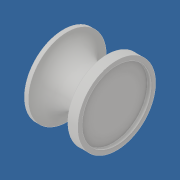
# Autodesk Inventor part: Brennersockel
Saved by Autodesk Inventor 2018 (Build 220112000, 112)
## iProperties
Created: 2018-10-20
Part Number: Brennersockel
Material: Generisch
Document SubType Name: Modeling
Designer: M.Knabel
Density: 1 g/cm^3
Appearance: Vorgabe
Author: M.Knabel
Autodesk Inventor part; units mm, degrees
ref_plane "YZ Plane" through (0, 0, 0) normal (1, 0, 0) x (0, 1, 0)
ref_plane "XZ Plane" through (0, 0, 0) normal (0, 1, 0) x (-1, 0, 0)
ref_plane "XY Plane" through (0, 0, 0) normal (0, 0, 1) x (1, 0, 0)
sketch "Skizze1" plane through (0, 0, 0) normal (0, 0, 1) x (1, 0, 0)
  line L0 (-5.4, 0) -> (32.4, 0) projected
  line L1 (0, -3.95) -> (0, 23.7) projected
  line L2 (0, 0) -> (0, 19.75)
  line L3 (2, 19.75) -> (0, 19.75)
  arc A0 (2, 19.75) -> (22, 19.75) centre (12, 19.75) ccw
  line L4 (22, 19.75) -> (27, 19.75)
  line L5 (27, 19.75) -> (27, 17.5)
  line L6 (27, 17.5) -> (25, 17.5)
  line L7 (25, 17.5) -> (25, 0)
  line L8 (0, 0) -> (25, 0)
  dimension "d0" = 27
  dimension "d1" = 2
  dimension "d2" = 39.5
  dimension "d3" = 10
  dimension "d4" = 12
  dimension "d5" = 5
  dimension "d6" = 35
  constraints: 14 end point, 4 perpendicular, 2 collinear, 2 point on circle, 2 point on line, 1 centre point, 1 horizontal
  measures "d0" distance between parallel lines of L5 L1
  measures "d1" distance between parallel lines of L7 L5
  measures "d2" diameter of L3 L0
  measures "d3" radius of A0
  measures "d4" distance from line of A0.centre L2
  measures "d5" distance of L4.end L4.start
  measures "d6" diameter of L6 L0
revolve "Umdrehung1" add sketch "Skizze1" angle 360 about axis through (-10, 0, 0) along (1, 0, 0)
sketch "Skizze2" plane through (0, 0, 0) normal (-1, 0, 0) x (0, 0, 1)
  point P0 (0, 0)
  point P1 (0, 0)
  constraints: 1 coincident
hole "Bohrung1" at (0, 0, 0) direction (1, 0, 0) diameter 3.242 depth 16 tip angle 118 thread size "M4x0.7" class "6H" standard "ISO Metric profile"
